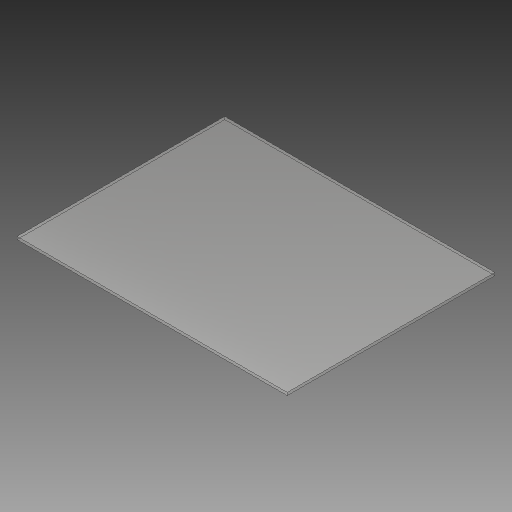
# Autodesk Inventor part: acrylic cover
Saved by Autodesk Inventor 2019 (Build 230136000, 136)
## iProperties
Created: 2019-06-26
Part Number: acrylic cover
Material: PMMA Plastic
Document SubType Name: Modeling
Designer: Daniel
Density: 1.188 g/cm^3
Appearance: Polycarbonate - Clear
Author: Daniel
Autodesk Inventor part; units mm, degrees
ref_plane "YZ Plane" through (0, 0, 0) normal (1, 0, 0) x (0, 1, 0)
ref_plane "XZ Plane" through (0, 0, 0) normal (0, 1, 0) x (-1, 0, 0)
ref_plane "XY Plane" through (0, 0, 0) normal (0, 0, 1) x (1, 0, 0)
sketch "Sketch1" plane through (0, 0, 0) normal (0, 1, 0) x (-1, 0, 0)
  line L0 (-120.4831, 80.3292) -> (4.5395, 80.3292)
  line L1 (4.5395, 80.3292) -> (4.5395, -15.7906)
  line L2 (4.5395, -15.7906) -> (-120.4831, -15.7906)
  line L3 (-120.4831, -15.7906) -> (-120.4831, 80.3292)
  point P0 (0, 0)
  constraints: 8 end point, 2 parallel, 1 horizontal, 1 perpendicular
extrude "Extrusion1" add sketch "Sketch1" along normal blind 1.27
body "Solid1"
